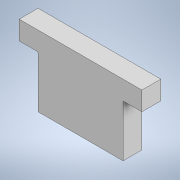
# Autodesk Inventor part: Tapa_1_TFM
Saved by Autodesk Inventor 2021 (Build 250183000, 183)
## iProperties
Created: 2023-07-25
Part Number: Tapa_1_TFM
Material: Generic
Document SubType Name: Modeling
Designer: alu01
Density: 1 g/cm^3
Appearance: Default
Author: alu01
Autodesk Inventor part; units mm, degrees
ref_plane "YZ Plane" through (0, 0, 0) normal (1, 0, 0) x (0, 1, 0)
ref_plane "XZ Plane" through (0, 0, 0) normal (0, 1, 0) x (-1, 0, 0)
ref_plane "XY Plane" through (0, 0, 0) normal (0, 0, 1) x (1, 0, 0)
sketch "Sketch1" plane through (0, 0, 0) normal (0, 0, 1) x (1, 0, 0)
  line L0 (4.5, -3.75) -> (-4.5, -3.75)
  line L1 (-4.5, -3.75) -> (-4.5, 3.75)
  line L2 (-4.5, 3.75) -> (4.5, 3.75)
  line L3 (4.5, 3.75) -> (4.5, -3.75)
  line L4 (4.5, -3.75) -> (-4.5, 3.75) construction
  line L5 (-4.5, -3.75) -> (4.5, 3.75) construction
  point P0 (0, 0)
  dimension "d0" = 9
  dimension "d1" = 7.5
  constraints: 12 end point, 2 midpoint, 2 parallel, 1 horizontal, 1 perpendicular
  measures "d0" distance of L1.end L2.end
  measures "d1" distance of L0.end L1.end
extrude "Extrusion1" add sketch "Sketch1" along normal mid plane 2
sketch "Sketch2" plane through (4.5, -3.75, 1) normal (1, 0, 0) x (0, 0, -1)
  line L0 (2, 7.5) -> (0, 7.5) projected
  line L1 (2, 7.5) -> (0, 7.5)
  line L2 (0, 7.5) -> (0, 5.5)
  line L3 (0, 5.5) -> (2, 5.5)
  line L4 (2, 5.5) -> (2, 7.5)
  point P0 (1, 3.75)
  dimension "d4" = 2
  dimension "d5" = 2
  constraints: 8 end point, 2 parallel, 1 horizontal, 1 perpendicular
  measures "d4" distance of L3.end L2.end
  measures "d5" distance of L1.end L2.end
extrude "Extrusion2" add sketch "Sketch2" along normal blind 2
sketch "Sketch3" plane through (-4.5, -3.75, 1) normal (-1, 0, 0) x (0, 0, 1)
  line L0 (-2, 7.5) -> (0, 7.5) projected
  line L1 (0, 7.5) -> (0, 0) projected
  line L2 (-2, 7.5) -> (0, 7.5)
  line L3 (0, 7.5) -> (0, 5.5)
  line L4 (0, 5.5) -> (-2, 5.5)
  line L5 (-2, 5.5) -> (-2, 7.5)
  point P0 (-1, 3.75)
  dimension "d8" = 2
  constraints: 8 end point, 2 parallel, 1 horizontal, 1 perpendicular, 1 point on line
  measures "d8" distance of L4.end L0.start
extrude "Extrusion3" add sketch "Sketch3" along normal blind 2
fillet "Fillet1" radius 0.1 2 edges at (4.5, 1.75, 0) (-4.5, 1.75, 0)
body "Solid1"
